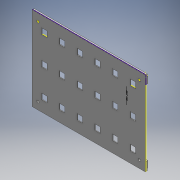
# Autodesk Inventor part: portaled
Saved by Autodesk Inventor 2016 (Build 200138000, 138)
## iProperties
Created: 2017-11-13
Part Number: portaled
Material: Generic
Document SubType Name: Modeling
Designer: Davide
Density: 1 g/cm^3
Appearance: Default
Author: Davide
Autodesk Inventor part; units mm, degrees
ref_plane "YZ Plane" through (0, 0, 0) normal (1, 0, 0) x (0, 1, 0)
ref_plane "XZ Plane" through (0, 0, 0) normal (0, 1, 0) x (-1, 0, 0)
ref_plane "XY Plane" through (0, 0, 0) normal (0, 0, 1) x (1, 0, 0)
sketch "Sketch1" plane through (0, 0, 0) normal (0, 1, 0) x (-1, 0, 0)
  line L0 (54, 40) -> (-54, 40)
  line L1 (-54, 40) -> (-54, -40)
  line L2 (-54, -40) -> (54, -40)
  line L3 (54, -40) -> (54, 40)
  line L4 (44.85, 29.7) -> (39.65, 29.7)
  line L5 (39.65, 29.7) -> (39.65, 24.3)
  line L6 (39.65, 24.3) -> (44.85, 24.3)
  line L7 (44.85, 24.3) -> (44.85, 29.7)
  line L8 (44.85, 2.7) -> (39.65, 2.7)
  line L9 (39.65, 2.7) -> (39.65, -2.7)
  line L10 (39.65, -2.7) -> (44.85, -2.7)
  line L11 (44.85, -2.7) -> (44.85, 2.7)
  line L12 (44.85, -24.3) -> (39.65, -24.3)
  line L13 (39.65, -24.3) -> (39.65, -29.7)
  line L14 (39.65, -29.7) -> (44.85, -29.7)
  line L15 (44.85, -29.7) -> (44.85, -24.3)
  line L16 (27.95, 29.7) -> (22.75, 29.7)
  line L17 (22.75, 29.7) -> (22.75, 24.3)
  line L18 (22.75, 24.3) -> (27.95, 24.3)
  line L19 (27.95, 24.3) -> (27.95, 29.7)
  line L20 (27.95, 2.7) -> (22.75, 2.7)
  line L21 (22.75, 2.7) -> (22.75, -2.7)
  line L22 (22.75, -2.7) -> (27.95, -2.7)
  line L23 (27.95, -2.7) -> (27.95, 2.7)
  line L24 (27.95, -24.3) -> (22.75, -24.3)
  line L25 (22.75, -24.3) -> (22.75, -29.7)
  line L26 (22.75, -29.7) -> (27.95, -29.7)
  line L27 (27.95, -29.7) -> (27.95, -24.3)
  line L28 (11.05, 29.7) -> (5.85, 29.7)
  line L29 (5.85, 29.7) -> (5.85, 24.3)
  line L30 (5.85, 24.3) -> (11.05, 24.3)
  line L31 (11.05, 24.3) -> (11.05, 29.7)
  line L32 (11.05, 2.7) -> (5.85, 2.7)
  line L33 (5.85, 2.7) -> (5.85, -2.7)
  line L34 (5.85, -2.7) -> (11.05, -2.7)
  line L35 (11.05, -2.7) -> (11.05, 2.7)
  line L36 (11.05, -24.3) -> (5.85, -24.3)
  line L37 (5.85, -24.3) -> (5.85, -29.7)
  line L38 (5.85, -29.7) -> (11.05, -29.7)
  line L39 (11.05, -29.7) -> (11.05, -24.3)
  line L40 (-5.85, 29.7) -> (-11.05, 29.7)
  line L41 (-11.05, 29.7) -> (-11.05, 24.3)
  line L42 (-11.05, 24.3) -> (-5.85, 24.3)
  line L43 (-5.85, 24.3) -> (-5.85, 29.7)
  line L44 (-5.85, 2.7) -> (-11.05, 2.7)
  line L45 (-11.05, 2.7) -> (-11.05, -2.7)
  line L46 (-11.05, -2.7) -> (-5.85, -2.7)
  line L47 (-5.85, -2.7) -> (-5.85, 2.7)
  line L48 (-5.85, -24.3) -> (-11.05, -24.3)
  line L49 (-11.05, -24.3) -> (-11.05, -29.7)
  line L50 (-11.05, -29.7) -> (-5.85, -29.7)
  line L51 (-5.85, -29.7) -> (-5.85, -24.3)
  line L52 (-22.75, 29.7) -> (-27.95, 29.7)
  line L53 (-27.95, 29.7) -> (-27.95, 24.3)
  line L54 (-27.95, 24.3) -> (-22.75, 24.3)
  line L55 (-22.75, 24.3) -> (-22.75, 29.7)
  line L56 (-22.75, 2.7) -> (-27.95, 2.7)
  line L57 (-27.95, 2.7) -> (-27.95, -2.7)
  line L58 (-27.95, -2.7) -> (-22.75, -2.7)
  line L59 (-22.75, -2.7) -> (-22.75, 2.7)
  line L60 (-22.75, -24.3) -> (-27.95, -24.3)
  line L61 (-27.95, -24.3) -> (-27.95, -29.7)
  line L62 (-27.95, -29.7) -> (-22.75, -29.7)
  line L63 (-22.75, -29.7) -> (-22.75, -24.3)
  line L64 (-39.65, 29.7) -> (-44.85, 29.7)
  line L65 (-44.85, 29.7) -> (-44.85, 24.3)
  line L66 (-44.85, 24.3) -> (-39.65, 24.3)
  line L67 (-39.65, 24.3) -> (-39.65, 29.7)
  line L68 (-39.65, 2.7) -> (-44.85, 2.7)
  line L69 (-44.85, 2.7) -> (-44.85, -2.7)
  line L70 (-44.85, -2.7) -> (-39.65, -2.7)
  line L71 (-39.65, -2.7) -> (-39.65, 2.7)
  line L72 (-39.65, -24.3) -> (-44.85, -24.3)
  line L73 (-44.85, -24.3) -> (-44.85, -29.7)
  line L74 (-44.85, -29.7) -> (-39.65, -29.7)
  line L75 (-39.65, -29.7) -> (-39.65, -24.3)
  line L76 (54, 0) -> (-54, 0) construction
  line L77 (0, 40) -> (0, -40) construction
  line L78 (5.85, 0) -> (-5.85, 0) construction
  circle A0 centre (48.35, 33) radius 1.1
  circle A1 centre (-48.35, 33) radius 1.1
  line L79 (48.35, 33) -> (-48.35, 33) construction
  circle A2 centre (48.35, -33) radius 1.1
  circle A3 centre (-48.35, -33) radius 1.1
  point P0 (0, 0)
  point P1 (44.85, 0)
  point P2 (0, 0)
  point P3 (0, 33)
  point P4 (0, 0)
  dimension "d0" = 108
  dimension "d1" = 80
  dimension "d2" = 5.2
  dimension "d3" = 5.4
  dimension "d6" = 27
  dimension "d9" = 16.9
  dimension "d12" = 2.2
  dimension "d13" = 2.2
  dimension "d14" = 96.7
  dimension "d15" = 33
  constraints: 160 end point, 11 midpoint, 5 horizontal, 4 centre point, 4 parallel, 4 point on line, 2 perpendicular, 2 symmetric about line, 1 coincident, 1 vertical, 138 other
  measures "d0" distance of L2.end L1.end
  measures "d1" distance of L0.end L1.end
  measures "d2" distance of L6.end L5.end
  measures "d3" distance of L5.end L4.end
  measures "d6" distance of L4.start L8.start
  measures "d9" distance of L4.start L16.start
  measures "d12" diameter of A1
  measures "d13" diameter of A0
  measures "d14" distance of L79.end L79.start
  measures "d15" distance between parallel lines of L76 L79
extrude "Extrusion1" add sketch "Sketch1" along normal blind 0.6
sketch "Sketch2" plane through (0, 0.6, 0) normal (0, 1, 0) x (1, 0, 0)
  line L0 (53.2, 0) -> (54, 0)
  line L1 (-53.2, 0) -> (-54, 0)
  line L2 (-44.85, -14.5) -> (44.85, -14.5)
  line L3 (44.85, -14.5) -> (44.85, -12.5)
  line L4 (44.85, -12.5) -> (-44.85, -12.5)
  line L5 (-44.85, -12.5) -> (-44.85, -14.5)
  line L6 (-44.85, -24.3) -> (-39.65, -24.3) projected
  line L7 (-39.65, -2.7) -> (-44.85, -2.7) projected
  line L8 (-44.85, -24.3) -> (-44.85, -2.7) construction
  line L9 (39.65, -24.3) -> (44.85, -24.3) projected
  line L10 (44.85, -2.7) -> (39.65, -2.7) projected
  line L11 (44.85, -24.3) -> (44.85, -2.7) construction
  line L12 (54, -31.9) -> (47.25, -31.9)
  line L13 (47.25, -31.9) -> (47.25, -38)
  line L14 (47.25, -38) -> (54, -38)
  line L15 (54, -38) -> (54, -31.9)
  circle A0 centre (48.35, -33) radius 1.1 projected
  circle A1 centre (-48.35, -33) radius 1.1 projected
  line L16 (-54, -38) -> (-47.25, -38)
  line L17 (-47.25, -38) -> (-47.25, -31.9)
  line L18 (-47.25, -31.9) -> (-54, -31.9)
  line L19 (-54, -31.9) -> (-54, -38)
  line L20 (54, -40) -> (54, 40) projected
  line L21 (-54, 40) -> (-54, -40) projected
  line L22 (-54, -40) -> (54, -40)
  line L23 (54, -40) -> (54, -38)
  line L24 (54, -38) -> (-54, -38)
  line L25 (-54, -38) -> (-54, -40)
  point P0 (0, 0)
  point P1 (54, -40)
  point P2 (-44.85, -13.5)
  point P3 (44.85, -13.5)
  dimension "d21" = 2
  constraints: 40 end point, 8 parallel, 5 perpendicular, 4 horizontal, 4 midpoint, 4 tangent, 2 point on line, 1 vertical
  measures "d21" distance between parallel lines of L4 L2
extrude "Extrusion2" add sketch "Sketch2" along normal blind 1.4 contours L5 L4 L3 L2 | L15 L14 L13 A0 L12 | A0 L13 L12 | L20 L22 L21 L16 L24 L14 | L16 L19 L18 A1 L17 | A1 L18 L17
mirror "Mirror1" about plane through (0, 0, 0) normal (0, 0, 1) of "Extrusion2"
extrude "Extrusion3" add sketch "Sketch2" along normal blind 2 contours L15 L14 L13 A0 L12 | A0 L13 L12 | L16 L19 L18 A1 L17 | A1 L18 L17
mirror "Mirror2" about plane through (0, 0, 0) normal (0, 0, 1) of "Extrusion3"
equation "\"d13\" = d12"
body "Solid1"
